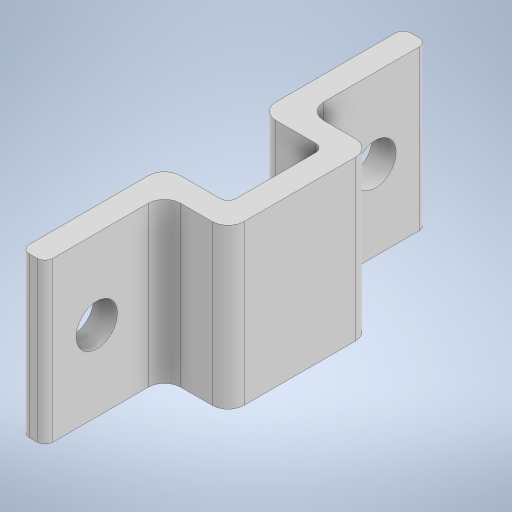
# Autodesk Inventor part: motor_clamp_v2
Saved by Autodesk Inventor 2024.2 (Build 282272000, 272)
## iProperties
Created: 2024-02-26
Part Number: motor_clamp_v2
Material: Ogólny
Document SubType Name: Modeling
Designer: Konrad
Density: 1 g/cm^3
Appearance: Domyślna
Author: Konrad
Autodesk Inventor part; units mm, degrees
ref_plane "YZ Plane" through (0, 0, 0) normal (1, 0, 0) x (0, 1, 0)
ref_plane "XZ Plane" through (0, 0, 0) normal (0, 1, 0) x (-1, 0, 0)
ref_plane "XY Plane" through (0, 0, 0) normal (0, 0, 1) x (1, 0, 0)
sketch "Szkic1" plane through (0, 0, 0) normal (0, 1, 0) x (-1, 0, 0)
  line L0 (0, 0) -> (0, -18)
  line L1 (0, -18) -> (-8, -18)
  line L2 (-8, -18) -> (-8, -30)
  line L3 (-8, -30) -> (0, -30)
  line L4 (0, -30) -> (0, -48)
  line L5 (0, -48) -> (-3, -48)
  line L6 (-3, -48) -> (-3, -33)
  line L7 (-3, -33) -> (-11, -33)
  line L8 (-11, -33) -> (-11, -15)
  line L9 (-11, -15) -> (-3, -15)
  line L10 (-3, -15) -> (-3, 0)
  line L11 (-3, 0) -> (0, 0)
  dimension "d0" = 48
  dimension "d2" = 8
  dimension "d3" = 12
  dimension "d4" = 3
  dimension "d5" = 3
  dimension "d6" = 3
  constraints: 24 end point, 10 perpendicular, 3 equal length, 2 point on line, 1 vertical
  measures "d0" distance of L4.end L0.start
  measures "d2" distance of L0.end L1.end
  measures "d3" distance of L1.end L2.end
  measures "d4" distance of L10.end L0.start
  measures "d5" distance between parallel lines of L1 L9
  measures "d6" distance between parallel lines of L8 L2
extrude "Wyciągnięcie proste1" add sketch "Szkic1" along normal blind 20
fillet "Zaokrąglenie1" radius 2 6 edges at (11, 10, -15) (3, 10, -15) (11, 10, -33) (3, 10, -33) (0, 10, -18) (0, 10, -30)
fillet "Zaokrąglenie2" radius 1 6 edges at (3, 10, 0) (0, 10, 0) (0, 10, -48) (3, 10, -48) (8, 10, -30) (8, 10, -18)
sketch "Szkic2" plane through (0, 0, -32) normal (-1, 0, 0) x (0, 0, 1)
  line L0 (-15, 0) -> (-15, 20) projected
  line L1 (-15, 0) -> (0, 0) projected
  line L2 (0, 20) -> (0, 0) projected
  line L3 (-15, 20) -> (0, 20) projected
  line L4 (31, 20) -> (31, 0) projected
  line L5 (16, 20) -> (31, 20) projected
  line L6 (16, 0) -> (16, 20) projected
  line L7 (16, 0) -> (31, 0) projected
  line L8 (15, 0) -> (1, 0) projected
  line L9 (8, 0) -> (8, 20) construction
  line L10 (3, 20) -> (13, 20) projected
  circle A0 centre (-9.5, 10) radius 2.6
  circle A1 centre (25.5, 10) radius 2.6
  point P0 (32, 0)
  dimension "d11" = 5.2
  dimension "d13" = 10
  dimension "d14" = 35
  constraints: 2 centre point, 2 end point, 2 midpoint, 1 equal radius, 1 symmetric about line
  measures "d11" diameter of A0
  measures "d13" distance from line of L1 A0.centre
  measures "d14" distance of A1.centre A0.centre
extrude "Wyciągnięcie proste2" cut sketch "Szkic2" against normal up to surface (3 mm away) contours A0 | A1
